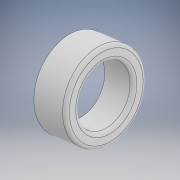
# Autodesk Inventor part: MuzzleWireProtector
Saved by Autodesk Inventor 2020.4 (Build 244396010, 396A)
## iProperties
Created: 2022-09-12
Part Number: MuzzleWireProtector
Material: Generic
Document SubType Name: Modeling
Designer: Val
Density: 1 g/cm^3
Appearance: Default
Author: Val
Autodesk Inventor part; units mm, degrees
ref_plane "YZ Plane" through (0, 0, 0) normal (1, 0, 0) x (0, 1, 0)
ref_plane "XZ Plane" through (0, 0, 0) normal (0, 1, 0) x (-1, 0, 0)
ref_plane "XY Plane" through (0, 0, 0) normal (0, 0, 1) x (1, 0, 0)
sketch "Base" plane through (0, 0, 0) normal (0, 0, 1) x (1, 0, 0)
  arc A0 (74.8, -14.5396) -> (75.632, 9.2864) centre (0, 0) ccw construction
  line L0 (0, 0) -> (69.0607, 32.2035) construction
  line L1 (0, 0) -> (74.8, -14.5396) construction
  line L2 (0, 0) -> (0, 77.8865) construction
  arc A1 (4.4887, 76.677) -> (0, 77.8865) centre (-17.0516, 5.6724) ccw construction
  arc A2 (74.8, -14.5396) -> (69.0607, 32.2035) centre (0, 0) ccw
  line L3 (69.0607, 32.2035) -> (74.8, -14.5396) construction
  line L4 (74.8, -14.5396) -> (93.708, -12.218)
  line L5 (93.708, -12.218) -> (90.8383, 11.1535)
  line L6 (87.9687, 34.5251) -> (69.0607, 32.2035) construction
  line L7 (90.8383, 11.1535) -> (71.9303, 8.8319) construction
  line L8 (90.8383, 11.1535) -> (87.9687, 34.5251) construction
  arc A3 (75.632, 9.2864) -> (27.6209, 71.0178) centre (0, 0) ccw construction
  line L9 (90.8383, 11.1535) -> (75.632, 9.2864)
  point P0 (0, 0)
  point P1 (75.632, 9.2864)
  dimension "d0" = 65
  dimension "d1" = 36
  dimension "d10" = 76.2
  dimension "d11" = 19.05
  constraints: 20 end point, 12 point on circle, 4 centre point, 3 parallel, 2 perpendicular, 2 point on line, 1 coincident, 1 collinear, 1 concentric, 1 midpoint, 1 vertical
  measures "d0" angle of L2 L0
  measures "d1" angle of L1 L0
  measures "d10" radius of A0
  measures "d11" distance of L4.end L1.end
revolve "BaseFeature" add sketch "Base" angle 360 about axis through (90.8383, 11.1535, 0) along (-0.9925462, -0.1218693, 0)
sketch "Hole" plane through (90.8383, 11.1535, 0) normal (0.9925462, 0.1218693, 0) x (0, 0, -1)
  circle A0 centre (0, 0) radius 15.875
  point P0 (0, 0)
  dimension "d13" = 31.75
  constraints: 1 centre point, 1 coincident
  measures "d13" diameter of A0
extrude "HoleFeature" cut sketch "Hole" against normal blind 25.4
fillet "FilletsFeature" radius 2 2 edges at (90.8383, 11.1535, 15.875) (87.9687, 34.5251, 0)
body "Solid2"
